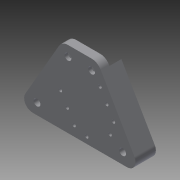
# Autodesk Inventor part: joint2+ax12print
Saved by Autodesk Inventor 2014 (Build 180170000, 170)
## iProperties
Created: 2014-01-12
Part Number: joint2+ax12print
Material: Générique
Document SubType Name: Modeling
Designer: helly
Density: 1 g/cm^3
Appearance: Par défaut
d1: 73,000 mm
d2: 60,00 deg
d3: 45,000 mm
d5: 39,000 mm
d7: 7,000 mm
d17: 6,500 mm
d18: 7,500 mm
d20: 4,000 mm
d21: 12,000 mm
d22: 0,00 deg
d23: 60,00 deg
d24: 13,500 mm
d25: 6,500 mm
d26: 8,000 mm
d27: 8,000 mm
d28: 8,000 mm
d30: 36,000 mm
d31: 8,000 mm
d32: 2,000 mm
d34: 0,00 deg
d35: 7,000 mm
d36: 3,000 mm
d37: 0,00 deg
d38: 12,000 mm
d43: 7,000 mm
d44: 0,00 deg
d45: 3,000 mm
d46: 0,00 deg
d48: 11,000 mm
d49: 6,000 mm
d50: 6,000 mm
d51: 5,000 mm
d52: 5,000 mm
Author: helly
Autodesk Inventor part; units mm, degrees
ref_plane "YZ Plane" through (0, 0, 0) normal (1, 0, 0) x (0, 1, 0)
ref_plane "XZ Plane" through (0, 0, 0) normal (0, 1, 0) x (-1, 0, 0)
ref_plane "XY Plane" through (0, 0, 0) normal (0, 0, 1) x (1, 0, 0)
sketch "Esquisse1" plane through (0, 0, 0) normal (0, 1, 0) x (-1, 0, 0)
  line L0 (0, 0) -> (73, 0) construction
  line L1 (73, 0) -> (36.5, 63.2199) construction
  line L2 (36.5, 63.2199) -> (0, 0) construction
  line L3 (0, 0) -> (0, 45) construction
  line L4 (0, 45) -> (25.9808, 45) construction
  line L5 (73, 0) -> (73, 39) construction
  line L6 (73, 39) -> (50.4833, 39) construction
  line L7 (22.5167, 39) -> (29.5167, 39) construction
  line L8 (50.4833, 39) -> (43.4833, 39) construction
  line L9 (25.9808, 45) -> (47.0192, 45) construction
  line L10 (43.4833, 45) -> (43.4833, 39) construction
  line L11 (29.5167, 39) -> (29.5167, 45) construction
  line L12 (3.7528, 6.5) -> (11.2528, 6.5) construction
  line L13 (11.2528, 6.5) -> (11.2528, 0) construction
  line L14 (73, 0) -> (73, 6.5) construction
  line L15 (69.2472, 6.5) -> (61.7472, 6.5) construction
  line L16 (61.7472, 6.5) -> (61.7472, 0) construction
  circle A0 centre (29.5167, 39) radius 2
  circle A1 centre (43.4833, 39) radius 2
  circle A2 centre (11.2528, 6.5) radius 2
  circle A3 centre (61.7472, 6.5) radius 2
  line L17 (0, 0) -> (73, 0)
  line L18 (47.0192, 45) -> (73, 0)
  line L19 (47.0192, 45) -> (25.9808, 45)
  line L20 (25.9808, 45) -> (0, 0)
  dimension "d1" = 73
  dimension "d2" = 60
  dimension "d3" = 45
  dimension "d5" = 39
  dimension "d7" = 7
  dimension "d17" = 6.5
  dimension "d18" = 7.5
  dimension "d20" = 4
  constraints: 42 end point, 11 perpendicular, 10 point on line, 5 collinear, 5 equal length, 4 centre point, 4 coincident, 3 equal radius, 2 parallel, 1 horizontal
  measures "d1" distance of L0.end L1.end
  measures "d2" angle of L1 L0
  measures "d3" distance of L0.start L3.end
  measures "d5" distance of L0.end L5.end
  measures "d7" distance of L6.end L8.end
  measures "d17" distance of L12.end L13.end
  measures "d18" distance of L12.start L12.end
  measures "d20" diameter of A0
extrude "Extrusion1" add sketch "Esquisse1" along normal blind 12
sketch "Esquisse2" plane through (0, 12, 0) normal (0, 1, 0) x (1, 0, 0)
  circle A0 centre (-43.4833, -39) radius 2 projected
  line L0 (0, 0) -> (-73, 0) projected
  line L1 (-47.0192, -45) -> (-21.0385, 0) construction
  line L2 (-47.0192, -45) -> (4.9423, -45) construction
  line L3 (-43.4833, -39) -> (-55.1747, -32.25) construction
  line L4 (-55.1747, -32.25) -> (-51.9247, -26.6208) construction
  line L5 (-51.9247, -26.6208) -> (-47.9247, -19.6926) construction
  line L6 (-47.9247, -19.6926) -> (-43.9247, -12.7644) construction
  line L7 (-43.9247, -12.7644) -> (-39.9247, -5.8362) construction
  line L8 (-43.4833, -39) -> (-25.4833, -7.8231) construction
  line L9 (-25.4833, -7.8231) -> (-32.4115, -3.8231) construction
  circle A1 centre (-32.4115, -3.8231) radius 1
  circle A2 centre (-39.9247, -5.8362) radius 1
  circle A3 centre (-43.9247, -12.7644) radius 1
  circle A4 centre (-47.9247, -19.6926) radius 1
  circle A5 centre (-18.6628, -11.7609) radius 1
  circle A6 centre (-16.6497, -19.274) radius 1
  circle A7 centre (-20.6497, -26.2023) radius 1
  circle A8 centre (-24.6497, -33.1305) radius 1
  dimension "d23" = 60
  dimension "d24" = 13.5
  dimension "d25" = 6.5
  dimension "d26" = 8
  dimension "d27" = 8
  dimension "d28" = 8
  dimension "d30" = 36
  dimension "d31" = 8
  dimension "d32" = 2
  constraints: 18 end point, 8 centre point, 4 coincident, 4 perpendicular, 4 symmetric about line, 3 collinear, 3 equal radius, 1 equal length, 1 horizontal, 1 point on line, 4 other
  measures "d23" angle of L2 L1
  measures "d24" distance of L3.start L3.end
  measures "d25" distance of L3.end L4.end
  measures "d26" distance of L4.end L5.end
  measures "d27" distance of L5.end L6.end
  measures "d28" distance of L6.end L7.end
  measures "d30" distance of L3.start L8.end
  measures "d31" distance of L8.end L9.end
  measures "d32" diameter of A1
extrude "Extrusion2" cut sketch "Esquisse2" against normal through all contours A1 | A2 | A3 | A4 | A5 | A6 | A7 | A8
sketch "Esquisse3" plane through (0, 12, 0) normal (0, 1, 0) x (1, 0, 0)
  circle A0 centre (-61.7472, -6.5) radius 2 projected
  circle A1 centre (-11.2528, -6.5) radius 2 projected
  line L0 (0, 0) -> (-73, 0) projected
  line L1 (-57.7058, -6.5) -> (-59.7265, -10)
  line L2 (-59.7265, -10) -> (-63.7679, -10)
  line L3 (-63.7679, -10) -> (-65.7887, -6.5)
  line L4 (-65.7887, -6.5) -> (-63.7679, -3)
  line L5 (-63.7679, -3) -> (-59.7265, -3)
  line L6 (-59.7265, -3) -> (-57.7058, -6.5)
  line L7 (-15.2942, -6.5) -> (-13.2735, -3)
  line L8 (-13.2735, -3) -> (-9.2321, -3)
  line L9 (-9.2321, -3) -> (-7.2113, -6.5)
  line L10 (-7.2113, -6.5) -> (-9.2321, -10)
  line L11 (-9.2321, -10) -> (-13.2735, -10)
  line L12 (-13.2735, -10) -> (-15.2942, -6.5)
  line L13 (-59.7265, -3) -> (-59.7265, -10) construction
  circle A2 centre (-43.4833, -39) radius 2 projected
  circle A3 centre (-29.5167, -39) radius 2 projected
  line L14 (-47.0192, -45) -> (-25.9808, -45) projected
  line L15 (-33.5581, -39) -> (-31.5374, -35.5) construction
  line L16 (-31.5374, -35.5) -> (-27.4959, -35.5) construction
  line L17 (-27.4959, -35.5) -> (-25.4752, -39) construction
  line L18 (-25.4752, -39) -> (-27.4959, -42.5) construction
  line L19 (-27.4959, -42.5) -> (-31.5374, -42.5) construction
  line L20 (-31.5374, -42.5) -> (-33.5581, -39) construction
  line L21 (-39.4419, -39) -> (-41.4626, -42.5) construction
  line L22 (-41.4626, -42.5) -> (-45.5041, -42.5) construction
  line L23 (-45.5041, -42.5) -> (-47.5248, -39) construction
  line L24 (-47.5248, -39) -> (-45.5041, -35.5) construction
  line L25 (-45.5041, -35.5) -> (-41.4626, -35.5) construction
  line L26 (-41.4626, -35.5) -> (-39.4419, -39) construction
  dimension "d35" = 7
  constraints: 50 end point, 4 coincident, 4 parallel, 3 equal length, 1 perpendicular, 52 other
  measures "d35" distance of L5.end L1.end
extrude "Extrusion3" cut sketch "Esquisse3" against normal blind 3 contours L1 L2 L3 L4 L5 L6 | L7 L8 L9 L10 L11 L12
sketch "Esquisse4" plane through (0, 12, 0) normal (0, 1, 0) x (1, 0, 0)
  line L0 (-9.2321, -10) -> (-13.2735, -10) projected
  circle A0 centre (-43.4833, -39) radius 2 projected
  circle A1 centre (-29.5167, -39) radius 2 projected
  line L1 (-73, 0) -> (-47.0192, -45) projected
  line L2 (-47.0192, -45) -> (-25.9808, -45) projected
  line L3 (-25.9808, -45) -> (0, 0) projected
  circle A2 centre (-43.4833, -39) radius 12 construction
  line L4 (-25.4752, -39) -> (-27.4959, -42.5) construction
  line L5 (-27.4959, -42.5) -> (-31.5374, -42.5) construction
  line L6 (-31.5374, -42.5) -> (-33.5581, -39) construction
  line L7 (-33.5581, -39) -> (-31.5374, -35.5) construction
  line L8 (-31.5374, -35.5) -> (-27.4959, -35.5) construction
  line L9 (-27.4959, -35.5) -> (-25.4752, -39) construction
  line L10 (-17.0563, -42.7582) -> (-44.103, -23.9539) construction
  line L11 (-9.2321, -3) -> (-7.2113, -6.5) projected
  line L12 (-36.6332, -29.1473) -> (-27.4959, -35.5)
  line L13 (-27.4959, -35.5) -> (-23.9959, -41.5622)
  line L14 (-36.6332, -29.1473) -> (-78.0005, -0.3866) construction
  line L15 (-36.6332, -29.1473) -> (13.7496, -29.1473) construction
  line L16 (-7.2113, -6.5) -> (-9.2321, -10) projected
  circle A3 centre (-43.9247, -12.7644) radius 1 projected
  circle A4 centre (-47.9247, -19.6926) radius 1 projected
  line L17 (-43.9247, -12.7644) -> (-49.4247, -22.2907) construction
  spline S0 degree 3 poles (-69.2739, -6.4538) (-56.5582, -21.7262) (-45.89, -22.7115) (-36.6332, -29.1473) knots 0 0 0 0 1 1 1 1
  point P0 (-22.5009, -38.9728)
  dimension "d38" = 12
  dimension "d48" = 11
  constraints: 24 end point, 8 point on line, 3 parallel, 2 coincident, 2 collinear, 2 equal length, 1 horizontal, 21 other
  measures "d48" distance of L17.start L17.end
extrude "Extrusion4" cut sketch "Esquisse4" against normal blind 7 contours S0 L12 L13 L3 L2 L1
sketch "Esquisse5" plane through (0, 5, 0) normal (0, 1, 0) x (1, 0, 0)
  circle A0 centre (-29.5167, -39) radius 2 projected
  circle A1 centre (-43.4833, -39) radius 2 projected
  line L0 (-25.9808, -45) -> (-47.0192, -45) projected
  line L1 (-39.4419, -39) -> (-41.4626, -42.5)
  line L2 (-41.4626, -42.5) -> (-45.5041, -42.5)
  line L3 (-45.5041, -42.5) -> (-47.5248, -39)
  line L4 (-47.5248, -39) -> (-45.5041, -35.5)
  line L5 (-45.5041, -35.5) -> (-41.4626, -35.5)
  line L6 (-41.4626, -35.5) -> (-39.4419, -39)
  line L7 (-33.5581, -39) -> (-31.5374, -35.5)
  line L8 (-31.5374, -35.5) -> (-27.4959, -35.5)
  line L9 (-27.4959, -35.5) -> (-25.4752, -39)
  line L10 (-25.4752, -39) -> (-27.4959, -42.5)
  line L11 (-27.4959, -42.5) -> (-31.5374, -42.5)
  line L12 (-31.5374, -42.5) -> (-33.5581, -39)
  line L13 (-59.7265, -10) -> (-63.7679, -10) projected
  line L14 (-57.7058, -6.5) -> (-59.7265, -10) projected
  point P0 (0, 0)
  constraints: 24 end point, 3 equal length, 2 parallel, 1 coincident, 26 other
extrude "Extrusion5" cut sketch "Esquisse5" against normal blind 3
fillet "Congé1" radius 6 1 edges at (-25.9808, 2.5, 45)
fillet "Congé2" radius 6 1 edges at (-47.0192, 2.5, 45)
fillet "Congé3" radius 5 1 edges at (0, 6, 0)
fillet "Congé4" radius 5 1 edges at (-73, 6, 0)
